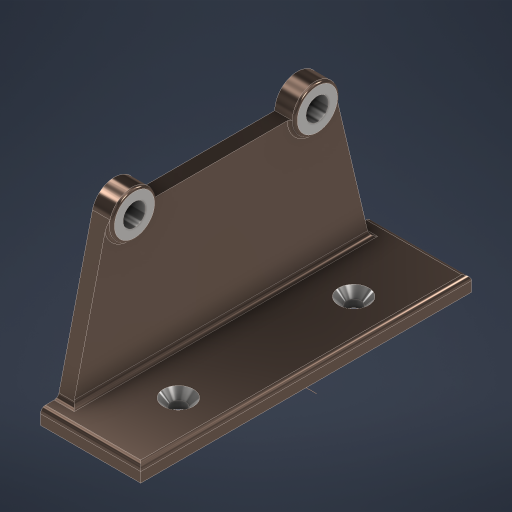
# Autodesk Inventor part: Support
Saved by Autodesk Inventor 2023 (Build 270158000, 158)
## iProperties
Created: 2022-11-28
Part Number: Support
Material: Steel
Document SubType Name: Modeling
Designer: iusti
Density: 7.85 g/cm^3
Appearance: Gunmetal - Antique Polished
Author: iusti
Autodesk Inventor part; units mm, degrees
ref_plane "YZ Plane" through (0, 0, 0) normal (1, 0, 0) x (0, 1, 0)
ref_plane "XZ Plane" through (0, 0, 0) normal (0, 1, 0) x (-1, 0, 0)
ref_plane "XY Plane" through (0, 0, 0) normal (0, 0, 1) x (1, 0, 0)
sketch "Sketch2" plane through (0, 0, 0) normal (0, 1, 0) x (-1, 0, 0)
  line L0 (0, 66) -> (-40, 66)
  line L1 (-40, 66) -> (-40, -66)
  line L2 (-40, -66) -> (0, -66)
  line L3 (0, -66) -> (0, 66)
  line L4 (-48, 0) -> (8, 0) construction
  point P0 (0, 0)
  dimension "d0" = 132
  dimension "d1" = 40
  constraints: 8 end point, 2 parallel, 1 horizontal, 1 midpoint, 1 perpendicular
  measures "d0" distance of L0.end L1.end
  measures "d1" distance of L1.end L2.end
extrude "Extrusion1" add sketch "Sketch2" along normal blind 6
sketch "Sketch3" plane through (0, 0, 0) normal (1, 0, 0) x (0, 1, 0)
  line L0 (0, 66) -> (0, -66) construction
  line L1 (6, 66) -> (6, -66) construction
  arc A0 (64.072464, -45.258133) -> (62, -27.5) centre (62, -36.5) ccw
  line L2 (-16.135746, 0) -> (96.814473, 0) construction
  line L3 (62, -27.5) -> (62, 0)
  line L4 (64.072464, -45.258133) -> (6, -59)
  arc A1 (62, 27.5) -> (64.072464, 45.258133) centre (62, 36.5) ccw
  line L5 (62, 27.5) -> (62, 0)
  line L6 (64.072464, 45.258133) -> (6, 59)
  line L7 (6, 59) -> (6, -59)
  point P0 (0, 0)
  point P1 (0, 0)
  dimension "d7" = 18
  dimension "d8" = 118
  dimension "d9" = 73
  dimension "d10" = 62
  constraints: 10 end point, 4 point on circle, 4 point on line, 4 symmetric about line, 2 centre point, 1 collinear, 1 midpoint, 1 perpendicular, 1 tangent, 1 other
  measures "d7" diameter of A0
  measures "d8" distance of L4.end L6.end
  measures "d9" distance of A0.centre A1.centre
  measures "d10" distance from line of L0 A0.centre
extrude "Extrusion2" add sketch "Sketch3" along normal blind 6
sketch "Sketch4" plane through (6, 0, 0) normal (1, 0, 0) x (0, 0, -1)
  arc A0 (45.258133, 64.072464) -> (27.5, 62) centre (36.5, 62) ccw
  arc A1 (-27.5, 62) -> (-45.258133, 64.072464) centre (-36.5, 62) ccw
  circle A2 centre (-36.5, 62) radius 9
  line L0 (27.5, 62) -> (-27.5, 62)
  circle A3 centre (36.5, 62) radius 9
  point P0 (0, 0)
  constraints: 2 coincident, 6 other
extrude "Extrusion3" add sketch "Sketch4" along normal blind 2
sketch "Sketch5" plane through (8, 62, 36.5) normal (1, 0, 0) x (0, 0, -1)
  circle A0 centre (0, 0) radius 9 projected
  circle A1 centre (73, 0) radius 9 projected
  point P0 (36.5, -62)
  constraints: 2 coincident
hole "Hole1" at (8, 62, 36.5) at (8, 62, -36.5) direction (-1, 0, 0) diameter 9 end through all
sketch "Sketch6" plane through (0, 6, 0) normal (0, 1, 0) x (1, 0, 0)
  line L0 (24, 35) -> (24, -35) construction
  line L1 (-8, 0) -> (48, 0) construction
  line L2 (0, 66) -> (0, -66) construction
  point P0 (0, 0)
  point P1 (24, 0)
  dimension "d22" = 70
  dimension "d23" = 24
  constraints: 2 coincident, 2 end point, 1 midpoint, 1 point on line, 1 vertical
  measures "d22" distance of L0.start L0.end
  measures "d23" distance from line of point (24, -35) L2
hole "Hole2" at (24, 6, -35) at (24, 6, 35) direction (0, -1, 0) diameter 6 end through all countersink diameter 12 countersink angle 90
fillet "Fillet1" radius 2 6 edges at (3, 6, 59) (20, 6, 66) (40, 6, 0) (20, 6, -66) (3, 6, -59) (6, 6, 0)
fillet "Fillet2" radius 1 4 edges at (8, 62, 45.5) (6, 53.0607, 37.5433) (8, 59.9275, -27.7419) (6, 53.0607, -37.5433)
body "Solid1"
